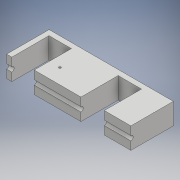
# Autodesk Inventor part: Arm_BaseV2
Saved by Autodesk Inventor 2017 (Build 210142000, 142)
## iProperties
Created: 2016-12-31
Part Number: Arm_BaseV2
Material: Generic
Document SubType Name: Modeling
Designer: Samanth
Density: 1 g/cm^3
Appearance: Default
Author: Samanth
Autodesk Inventor part; units mm, degrees
ref_plane "YZ Plane" through (0, 0, 0) normal (1, 0, 0) x (0, 1, 0)
ref_plane "XZ Plane" through (0, 0, 0) normal (0, 1, 0) x (-1, 0, 0)
ref_plane "XY Plane" through (0, 0, 0) normal (0, 0, 1) x (1, 0, 0)
sketch "Sketch1" plane through (0, 0, 0) normal (0, 0, 1) x (1, 0, 0)
  line L0 (0, 0) -> (68, 0)
  line L1 (68, 0) -> (68, 70)
  line L2 (68, 80) -> (112, 80)
  line L3 (112, 70) -> (112, 0)
  line L4 (112, 0) -> (162, 0)
  line L5 (162, 0) -> (162, 80)
  line L6 (162, 80) -> (68, 80)
  line L7 (68, 70) -> (112, 70)
  line L8 (68, 80) -> (-17, 80)
  line L9 (-17, 80) -> (-63, 80)
  line L10 (-63, 80) -> (-72, 80)
  line L11 (-72, 80) -> (-72, 0)
  line L12 (-72, 0) -> (-62.245, 0)
  line L13 (0, 0) -> (-17, 0)
  line L14 (-20.0216, 70) -> (-62.245, 70)
  line L15 (-20.0216, 70) -> (-20.0216, 0)
  line L16 (-20.0216, 0) -> (-17, 0)
  circle A0 centre (0, 28.3486) radius 2
  line L17 (-62.245, 0) -> (-62.245, 70)
  line L18 (-20.0216, 0) -> (68, 0)
  dimension "d6" = 46
  dimension "d7" = 9
  dimension "d8" = 4
  constraints: 38 end point, 7 perpendicular, 6 horizontal, 3 vertical, 2 point on line, 1 centre point
  measures "d6" distance of L8.end L9.end
  measures "d7" distance of L9.end L10.end
  measures "d8" diameter of A0
extrude "Extrusion1" add sketch "Sketch1" along normal mid plane 40
sketch "Sketch2" plane through (162, 0, 20) normal (1, 0, 0) x (0, 0, -1)
  circle A0 centre (20, 0) radius 4.4
  dimension "d11" = 8.8
  constraints: 1 centre point, 1 coincident
  measures "d11" diameter of A0
extrude "Extrusion2" cut sketch "Sketch2" against normal blind 1600
body "Solid1"
